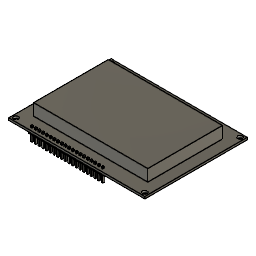
LCD_128x64-21M_V1.5 (Autodesk Fusion 360 design; units mm, degrees)
Autodesk Fusion 360 part; units mm, degrees
sketch "Sketch1" plane through (0, 0, 0) normal (0, 0, 1) x (1, 0, 0)
  circle A0 centre (2.5, -2.5) radius 1.6
  circle A1 centre (90.5, -2.5) radius 1.6
  circle A2 centre (2.5, -67.5) radius 1.6
  circle A3 centre (90.5, -67.5) radius 1.6
  line L0 (0, 0) -> (93, 0)
  line L1 (93, 0) -> (93, -70)
  line L2 (93, -70) -> (0, -70)
  line L3 (0, -70) -> (0, 0)
  line L4 (14.75, -68.75) -> (12.25, -68.75)
  line L5 (12.25, -68.75) -> (12.25, -66.25)
  line L6 (12.25, -66.25) -> (14.75, -66.25)
  line L7 (14.75, -66.25) -> (14.75, -68.75)
  line L8 (14.75, -68.75) -> (12.25, -66.25) construction
  line L9 (12.25, -68.75) -> (14.75, -66.25) construction
  line L10 (14.79, -68.75) -> (17.29, -66.25) construction
  line L11 (17.29, -68.75) -> (14.79, -66.25) construction
  line L12 (17.29, -66.25) -> (17.29, -68.75)
  line L13 (14.79, -66.25) -> (17.29, -66.25)
  line L14 (17.29, -68.75) -> (14.79, -68.75)
  line L15 (14.79, -68.75) -> (14.79, -66.25)
  line L16 (17.33, -68.75) -> (19.83, -66.25) construction
  line L17 (19.83, -68.75) -> (17.33, -66.25) construction
  line L18 (19.83, -66.25) -> (19.83, -68.75)
  line L19 (17.33, -66.25) -> (19.83, -66.25)
  line L20 (19.83, -68.75) -> (17.33, -68.75)
  line L21 (17.33, -68.75) -> (17.33, -66.25)
  line L22 (19.87, -68.75) -> (22.37, -66.25) construction
  line L23 (22.37, -68.75) -> (19.87, -66.25) construction
  line L24 (22.37, -66.25) -> (22.37, -68.75)
  line L25 (19.87, -66.25) -> (22.37, -66.25)
  line L26 (22.37, -68.75) -> (19.87, -68.75)
  line L27 (19.87, -68.75) -> (19.87, -66.25)
  line L28 (22.41, -68.75) -> (24.91, -66.25) construction
  line L29 (24.91, -68.75) -> (22.41, -66.25) construction
  line L30 (24.91, -66.25) -> (24.91, -68.75)
  line L31 (22.41, -66.25) -> (24.91, -66.25)
  line L32 (24.91, -68.75) -> (22.41, -68.75)
  line L33 (22.41, -68.75) -> (22.41, -66.25)
  line L34 (24.95, -68.75) -> (27.45, -66.25) construction
  line L35 (27.45, -68.75) -> (24.95, -66.25) construction
  line L36 (27.45, -66.25) -> (27.45, -68.75)
  line L37 (24.95, -66.25) -> (27.45, -66.25)
  line L38 (27.45, -68.75) -> (24.95, -68.75)
  line L39 (24.95, -68.75) -> (24.95, -66.25)
  line L40 (27.49, -68.75) -> (29.99, -66.25) construction
  line L41 (29.99, -68.75) -> (27.49, -66.25) construction
  line L42 (29.99, -66.25) -> (29.99, -68.75)
  line L43 (27.49, -66.25) -> (29.99, -66.25)
  line L44 (29.99, -68.75) -> (27.49, -68.75)
  line L45 (27.49, -68.75) -> (27.49, -66.25)
  line L46 (30.03, -68.75) -> (32.53, -66.25) construction
  line L47 (32.53, -68.75) -> (30.03, -66.25) construction
  line L48 (32.53, -66.25) -> (32.53, -68.75)
  line L49 (30.03, -66.25) -> (32.53, -66.25)
  line L50 (32.53, -68.75) -> (30.03, -68.75)
  line L51 (30.03, -68.75) -> (30.03, -66.25)
  line L52 (32.57, -68.75) -> (35.07, -66.25) construction
  line L53 (35.07, -68.75) -> (32.57, -66.25) construction
  line L54 (35.07, -66.25) -> (35.07, -68.75)
  line L55 (32.57, -66.25) -> (35.07, -66.25)
  line L56 (35.07, -68.75) -> (32.57, -68.75)
  line L57 (32.57, -68.75) -> (32.57, -66.25)
  line L58 (35.11, -68.75) -> (37.61, -66.25) construction
  line L59 (37.61, -68.75) -> (35.11, -66.25) construction
  line L60 (37.61, -66.25) -> (37.61, -68.75)
  line L61 (35.11, -66.25) -> (37.61, -66.25)
  line L62 (37.61, -68.75) -> (35.11, -68.75)
  line L63 (35.11, -68.75) -> (35.11, -66.25)
  line L64 (37.65, -68.75) -> (40.15, -66.25) construction
  line L65 (40.15, -68.75) -> (37.65, -66.25) construction
  line L66 (40.15, -66.25) -> (40.15, -68.75)
  line L67 (37.65, -66.25) -> (40.15, -66.25)
  line L68 (40.15, -68.75) -> (37.65, -68.75)
  line L69 (37.65, -68.75) -> (37.65, -66.25)
  line L70 (40.19, -68.75) -> (42.69, -66.25) construction
  line L71 (42.69, -68.75) -> (40.19, -66.25) construction
  line L72 (42.69, -66.25) -> (42.69, -68.75)
  line L73 (40.19, -66.25) -> (42.69, -66.25)
  line L74 (42.69, -68.75) -> (40.19, -68.75)
  line L75 (40.19, -68.75) -> (40.19, -66.25)
  line L76 (42.73, -68.75) -> (45.23, -66.25) construction
  line L77 (45.23, -68.75) -> (42.73, -66.25) construction
  line L78 (45.23, -66.25) -> (45.23, -68.75)
  line L79 (42.73, -66.25) -> (45.23, -66.25)
  line L80 (45.23, -68.75) -> (42.73, -68.75)
  line L81 (42.73, -68.75) -> (42.73, -66.25)
  line L82 (45.27, -68.75) -> (47.77, -66.25) construction
  line L83 (47.77, -68.75) -> (45.27, -66.25) construction
  line L84 (47.77, -66.25) -> (47.77, -68.75)
  line L85 (45.27, -66.25) -> (47.77, -66.25)
  line L86 (47.77, -68.75) -> (45.27, -68.75)
  line L87 (45.27, -68.75) -> (45.27, -66.25)
  line L88 (47.81, -68.75) -> (50.31, -66.25) construction
  line L89 (50.31, -68.75) -> (47.81, -66.25) construction
  line L90 (50.31, -66.25) -> (50.31, -68.75)
  line L91 (47.81, -66.25) -> (50.31, -66.25)
  line L92 (50.31, -68.75) -> (47.81, -68.75)
  line L93 (47.81, -68.75) -> (47.81, -66.25)
  line L94 (50.35, -68.75) -> (52.85, -66.25) construction
  line L95 (52.85, -68.75) -> (50.35, -66.25) construction
  line L96 (52.85, -66.25) -> (52.85, -68.75)
  line L97 (50.35, -66.25) -> (52.85, -66.25)
  line L98 (52.85, -68.75) -> (50.35, -68.75)
  line L99 (50.35, -68.75) -> (50.35, -66.25)
  line L100 (52.89, -68.75) -> (55.39, -66.25) construction
  line L101 (55.39, -68.75) -> (52.89, -66.25) construction
  line L102 (55.39, -66.25) -> (55.39, -68.75)
  line L103 (52.89, -66.25) -> (55.39, -66.25)
  line L104 (55.39, -68.75) -> (52.89, -68.75)
  line L105 (52.89, -68.75) -> (52.89, -66.25)
  line L106 (55.43, -68.75) -> (57.93, -66.25) construction
  line L107 (57.93, -68.75) -> (55.43, -66.25) construction
  line L108 (57.93, -66.25) -> (57.93, -68.75)
  line L109 (55.43, -66.25) -> (57.93, -66.25)
  line L110 (57.93, -68.75) -> (55.43, -68.75)
  line L111 (55.43, -68.75) -> (55.43, -66.25)
  line L112 (57.97, -68.75) -> (60.47, -66.25) construction
  line L113 (60.47, -68.75) -> (57.97, -66.25) construction
  line L114 (60.47, -66.25) -> (60.47, -68.75)
  line L115 (57.97, -66.25) -> (60.47, -66.25)
  line L116 (60.47, -68.75) -> (57.97, -68.75)
  line L117 (57.97, -68.75) -> (57.97, -66.25)
  line L118 (60.51, -68.75) -> (63.01, -66.25) construction
  line L119 (63.01, -68.75) -> (60.51, -66.25) construction
  line L120 (63.01, -66.25) -> (63.01, -68.75)
  line L121 (60.51, -66.25) -> (63.01, -66.25)
  line L122 (63.01, -68.75) -> (60.51, -68.75)
  line L123 (60.51, -68.75) -> (60.51, -66.25)
  line L124 (7.5, -9.5) -> (85.5, -9.5)
  line L125 (85.5, -9.5) -> (85.5, -60.5)
  line L126 (85.5, -60.5) -> (7.5, -60.5)
  line L127 (7.5, -60.5) -> (7.5, -9.5)
  line L128 (14, -67) -> (13, -67)
  line L129 (13, -67) -> (13, -68)
  line L130 (13, -68) -> (14, -68)
  line L131 (14, -68) -> (14, -67)
  line L132 (14, -67) -> (13, -68) construction
  line L133 (13, -67) -> (14, -68) construction
  line L134 (15.54, -68) -> (16.54, -68)
  line L135 (15.54, -67) -> (15.54, -68)
  line L136 (16.54, -67) -> (15.54, -67)
  line L137 (16.54, -68) -> (16.54, -67)
  line L138 (18.08, -68) -> (19.08, -68)
  line L139 (18.08, -67) -> (18.08, -68)
  line L140 (19.08, -67) -> (18.08, -67)
  line L141 (19.08, -68) -> (19.08, -67)
  line L142 (20.62, -68) -> (21.62, -68)
  line L143 (20.62, -67) -> (20.62, -68)
  line L144 (21.62, -67) -> (20.62, -67)
  line L145 (21.62, -68) -> (21.62, -67)
  line L146 (23.16, -68) -> (24.16, -68)
  line L147 (23.16, -67) -> (23.16, -68)
  line L148 (24.16, -67) -> (23.16, -67)
  line L149 (24.16, -68) -> (24.16, -67)
  line L150 (25.7, -68) -> (26.7, -68)
  line L151 (25.7, -67) -> (25.7, -68)
  line L152 (26.7, -67) -> (25.7, -67)
  line L153 (26.7, -68) -> (26.7, -67)
  line L154 (28.24, -68) -> (29.24, -68)
  line L155 (28.24, -67) -> (28.24, -68)
  line L156 (29.24, -67) -> (28.24, -67)
  line L157 (29.24, -68) -> (29.24, -67)
  line L158 (30.78, -68) -> (31.78, -68)
  line L159 (30.78, -67) -> (30.78, -68)
  line L160 (31.78, -67) -> (30.78, -67)
  line L161 (31.78, -68) -> (31.78, -67)
  line L162 (33.32, -68) -> (34.32, -68)
  line L163 (33.32, -67) -> (33.32, -68)
  line L164 (34.32, -67) -> (33.32, -67)
  line L165 (34.32, -68) -> (34.32, -67)
  line L166 (35.86, -68) -> (36.86, -68)
  line L167 (35.86, -67) -> (35.86, -68)
  line L168 (36.86, -67) -> (35.86, -67)
  line L169 (36.86, -68) -> (36.86, -67)
  line L170 (38.4, -68) -> (39.4, -68)
  line L171 (38.4, -67) -> (38.4, -68)
  line L172 (39.4, -67) -> (38.4, -67)
  line L173 (39.4, -68) -> (39.4, -67)
  line L174 (40.94, -68) -> (41.94, -68)
  line L175 (40.94, -67) -> (40.94, -68)
  line L176 (41.94, -67) -> (40.94, -67)
  line L177 (41.94, -68) -> (41.94, -67)
  line L178 (43.48, -68) -> (44.48, -68)
  line L179 (43.48, -67) -> (43.48, -68)
  line L180 (44.48, -67) -> (43.48, -67)
  line L181 (44.48, -68) -> (44.48, -67)
  line L182 (46.02, -68) -> (47.02, -68)
  line L183 (46.02, -67) -> (46.02, -68)
  line L184 (47.02, -67) -> (46.02, -67)
  line L185 (47.02, -68) -> (47.02, -67)
  line L186 (48.56, -68) -> (49.56, -68)
  line L187 (48.56, -67) -> (48.56, -68)
  line L188 (49.56, -67) -> (48.56, -67)
  line L189 (49.56, -68) -> (49.56, -67)
  line L190 (51.1, -68) -> (52.1, -68)
  line L191 (51.1, -67) -> (51.1, -68)
  line L192 (52.1, -67) -> (51.1, -67)
  line L193 (52.1, -68) -> (52.1, -67)
  line L194 (53.64, -68) -> (54.64, -68)
  line L195 (53.64, -67) -> (53.64, -68)
  line L196 (54.64, -67) -> (53.64, -67)
  line L197 (54.64, -68) -> (54.64, -67)
  line L198 (56.18, -68) -> (57.18, -68)
  line L199 (56.18, -67) -> (56.18, -68)
  line L200 (57.18, -67) -> (56.18, -67)
  line L201 (57.18, -68) -> (57.18, -67)
  line L202 (58.72, -68) -> (59.72, -68)
  line L203 (58.72, -67) -> (58.72, -68)
  line L204 (59.72, -67) -> (58.72, -67)
  line L205 (59.72, -68) -> (59.72, -67)
  line L206 (61.26, -68) -> (62.26, -68)
  line L207 (61.26, -67) -> (61.26, -68)
  line L208 (62.26, -67) -> (61.26, -67)
  line L209 (62.26, -68) -> (62.26, -67)
  point P0 (13.5, -67.5)
  point P1 (16.04, -67.5)
  point P2 (18.58, -67.5)
  point P3 (21.12, -67.5)
  point P4 (23.66, -67.5)
  point P5 (26.2, -67.5)
  point P6 (28.74, -67.5)
  point P7 (31.28, -67.5)
  point P8 (33.82, -67.5)
  point P9 (36.36, -67.5)
  point P10 (38.9, -67.5)
  point P11 (41.44, -67.5)
  point P12 (43.98, -67.5)
  point P13 (46.52, -67.5)
  point P14 (49.06, -67.5)
  point P15 (51.6, -67.5)
  point P16 (54.14, -67.5)
  point P17 (56.68, -67.5)
  point P18 (59.22, -67.5)
  point P19 (61.76, -67.5)
  point P20 (7.5, -9.5)
  point P21 (13.5, -67.5)
  dimension "d1" = 3.2
  dimension "d2" = 3.2
  dimension "d3" = 3.2
  dimension "d4" = 3.2
  dimension "d5" = 93
  dimension "d6" = 70
  dimension "d7" = 2.5
  dimension "d8" = 2.5
  dimension "d11" = 2.54
  dimension "d12" = 0
  dimension "d15" = 78
  dimension "d16" = 51
  dimension "d17" = 1
  dimension "d18" = 1
  dimension "d21" = 2.54
  dimension "d22" = 0
  constraint horizontal L0
  constraint vertical L1
  constraint horizontal L2
  constraint vertical L3
  constraint coincident L0.start L3.end
  constraint horizontal L4
  constraint perpendicular L4 L5
  constraint parallel L4 L6
  constraint parallel L5 L7
  constraint horizontal L124
  constraint vertical L125
  constraint horizontal L126
  constraint vertical L127
  constraint coincident P20 L124.start
  constraint horizontal L128
  constraint perpendicular L128 L129
  constraint parallel L128 L130
  constraint parallel L129 L131
  constraint coincident L132 P21
  constraint coincident L133 P21
  constraint coincident P21 P0
  measures "d1" diameter of A0
  measures "d2" diameter of A1
  measures "d3" diameter of A2
  measures "d4" diameter of A3
  measures "d5" distance of L0.start L0.end
  measures "d6" distance of L0.start L2.end
  measures "d7" distance of L5.end L6.end
  measures "d8" distance of L4.end L5.end
  measures "d15" distance of P20 L124.end
  measures "d16" distance of P20 L126.end
  measures "d17" distance of L129.end L130.end
  measures "d18" distance of L128.end L129.end
extrude "Extrude1" add sketch "Sketch1" along normal blind 2 contours L4 L5 L6 L7 | L12 L13 L14 L15 | L18 L19 L20 L21 | L24 L25 L26 L27 | L30 L31 L32 L33 | L36 L37 L38 L39 | L42 L43 L44 L45 | L48 L49 L50 L51 | L54 L55 L56 L57 | L60 L61 L62 L63 | L66 L67 L68 L69 | L72 L73 L74 L75 | L78 L79 L80 L81 | L84 L85 L86 L87 | L90 L91 L92 L93 | L96 L97 L98 L99 | L102 L103 L104 L105 | L108 L109 L110 L111 | L114 L115 L116 L117 | L120 L121 L122 L123 makes body 1 at (40.44, -67.3333, 0) makes body 2 at (51.4333, -68.5, 0) makes body 3 at (62.76, -67.6667, 0) makes body 4 at (26.3667, -68.5, 0) makes body 5 at (16.2067, -68.5, 0) makes body 6 at (18.7467, -68.5, 0) makes body 7 at (29.74, -67.6667, 0) makes body 8 at (59.3867, -68.5, 0) makes body 9 at (48.8933, -68.5, 0) makes body 10 at (39.0667, -68.5, 0) makes body 11 at (44.1467, -68.5, 0) makes body 12 at (55.14, -67.6667, 0) makes body 13 at (33.9867, -68.5, 0) makes body 14 at (23.8267, -68.5, 0) makes body 15 at (14.5, -67.6667, 0) makes body 16 at (20.12, -67.3333, 0) makes body 17 at (31.4467, -68.5, 0) makes body 18 at (55.68, -67.3333, 0) makes body 19 at (47.52, -67.6667, 0) makes body 20 at (36.5267, -68.5, 0)
move_body "Move1" bodies 3 16 20 10 18 11 7 5 6 4 2 13 19 9 17 15 1 12 8 14 to x (1, 0, 0) y (0, 1, 0) z (0, 0, 1) at (0, 0, -1.5)
move_body "Move2" bodies 1 8 5 12 14 16 19 6 9 2 4 7 11 10 13 3 15 18 20 17 to x (1, 0, 0) y (0, 1, 0) z (0, 0, 1) at (0, 0, -2)
extrude "Extrude2" add sketch "Sketch1" along normal blind 1.5 separate body contours L0 L1 L2 L3 makes body 21
move_body "Move3" bodies 1 8 5 12 14 16 19 6 9 2 4 7 11 10 13 3 15 18 20 17 to x (1, 0, 0) y (0, 1, 0) z (0, 0, 1) at (0, 0, 1.5)
extrude "Extrude3" add sketch "Sketch1" along normal blind 9.5 contours L124 L125 L126 L127 bodies 21
extrude "Extrude5" add sketch "Sketch1" against normal blind 5 separate body contours L128 L129 L130 L131 | L134 L135 L136 L137 | L138 L139 L140 L141 | L142 L143 L144 L145 | L146 L147 L148 L149 | L150 L151 L152 L153 | L154 L155 L156 L157 | L158 L159 L160 L161 | L162 L163 L164 L165 | L166 L167 L168 L169 | L170 L171 L172 L173 | L174 L175 L176 L177 | L178 L179 L180 L181 | L182 L183 L184 L185 | L186 L187 L188 L189 | L190 L191 L192 L193 | L194 L195 L196 L197 | L198 L199 L200 L201 | L202 L203 L204 L205 | L206 L207 L208 L209 makes body 22 at (36.5267, -67, -1.6667) makes body 23 at (46.02, -67.3333, -1.6667) makes body 24 at (56.18, -67.3333, -1.6667) makes body 25 at (25.7, -67.3333, -1.6667) makes body 26 at (15.54, -67.3333, -1.6667) makes body 27 at (18.7467, -67, -1.6667) makes body 28 at (28.24, -67.3333, -1.6667) makes body 29 at (53.64, -67.3333, -1.6667) makes body 30 at (43.48, -67.3333, -1.6667) makes body 31 at (33.9867, -67, -1.6667) makes body 32 at (38.4, -67.3333, -1.6667) makes body 33 at (48.8933, -68, -1.6667) makes body 34 at (59.3867, -67, -1.6667) makes body 35 at (23.16, -67.3333, -1.6667) makes body 36 at (14, -67.6667, -1.6667) makes body 37 at (20.62, -67.3333, -1.6667) makes body 38 at (61.26, -67.3333, -1.6667) makes body 39 at (51.7667, -67, -1.6667) makes body 40 at (41.6067, -67, -1.6667) makes body 41 at (31.4467, -67, -1.6667)
move_body "Move4" bodies 22 26 25 24 23 29 30 39 40 41 32 35 34 31 37 28 27 33 36 38 to x (1, 0, 0) y (0, 1, 0) z (0, 0, 1) at (0, 0, -2)
extrude "Extrude6" add sketch "Sketch1" along normal blind 1.5 contours L4 L5 L6 L7 | L12 L13 L14 L15 | L18 L19 L20 L21 | L24 L25 L26 L27 | L30 L31 L32 L33 | L36 L37 L38 L39 | L42 L43 L44 L45 | L48 L49 L50 L51 | L54 L55 L56 L57 | L60 L61 L62 L63 | L66 L67 L68 L69 | L72 L73 L74 L75 | L78 L79 L80 L81 | L84 L85 L86 L87 | L90 L91 L92 L93 | L96 L97 L98 L99 | L102 L103 L104 L105 | L108 L109 L110 L111 | L114 L115 L116 L117 | L120 L121 L122 L123 bodies 1 22 23 24 25 26 27 28 29 30 31 32 33 34 35 36 37 38 39 41 2 3 4 5 6 7 8 9 10 11 12 13 14 15 16 17 18 19 20 21
move_face "OffsetFaces1" offset 4.5 20 faces at (53.9733, -67.3333, -2) (46.3533, -67.3333, -2) (18.7467, -67.3333, -2) (28.5733, -67.3333, -2) (36.5267, -67.3333, -2) (26.0333, -67.3333, -2) (15.8733, -67.3333, -2) (56.8467, -67.6667, -2) (61.5933, -67.3333, -2) (51.4333, -67.3333, -2) (41.2733, -67.3333, -2) (31.4467, -67.3333, -2) (13.3333, -67.3333, -2) (20.9533, -67.3333, -2) (23.4933, -67.3333, -2) (33.9867, -67.3333, -2) (49.2267, -67.6667, -2) (38.7333, -67.3333, -2) (43.8133, -67.3333, -2) (59.0533, -67.3333, -2) on bodies 22 23 24 25 26 27 28 29 30 31 32 33 34 35 36 37 38 39 40 41
equation "d27 = 1.5 mm + 8 mm"
